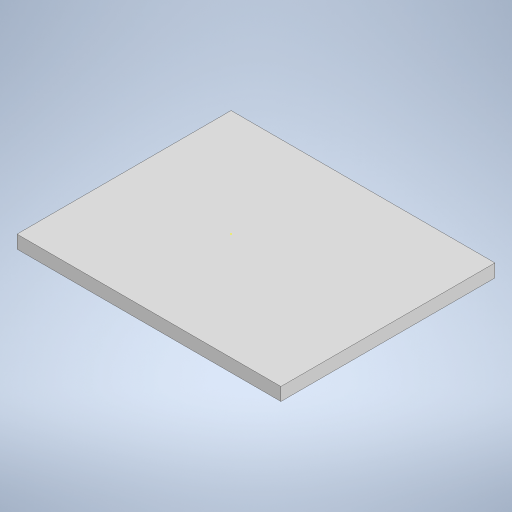
# Autodesk Inventor part: Base
Saved by Autodesk Inventor 2024 (Build 280153000, 153)
## iProperties
Created: 2023-10-07
Part Number: Base
Material: Generic
Document SubType Name: Modeling
Designer: chris
Density: 1 g/cm^3
Appearance: Default
Author: chris
Autodesk Inventor part; units mm, degrees
ref_plane "YZ Plane" through (0, 0, 0) normal (1, 0, 0) x (0, 1, 0)
ref_plane "XZ Plane" through (0, 0, 0) normal (0, 1, 0) x (-1, 0, 0)
ref_plane "XY Plane" through (0, 0, 0) normal (0, 0, 1) x (1, 0, 0)
sketch "Sketch1" plane through (0, 0, 0) normal (0, 1, 0) x (-1, 0, 0)
  line L0 (26.36, 26.36) -> (-26.36, 26.36)
  line L1 (-26.36, 26.36) -> (-26.36, -26.36)
  line L2 (-26.36, -26.36) -> (26.36, -26.36)
  line L3 (26.36, -26.36) -> (26.36, 26.36)
  line L4 (26.36, 26.36) -> (-26.36, -26.36) construction
  line L5 (-26.36, 26.36) -> (26.36, -26.36) construction
  line L6 (-26.36, -26.36) -> (-38.64, -26.36)
  line L7 (-38.64, -26.36) -> (-38.64, 26.36)
  line L8 (-38.64, 26.36) -> (-26.36, 26.36)
  line L9 (-26.36, 26.36) -> (-26.36, -26.36)
  point P0 (0, 0)
  dimension "d4" = 65
  dimension "d5" = 52.72
  constraints: 20 end point, 4 parallel, 3 perpendicular, 2 horizontal, 2 midpoint, 1 collinear
  measures "d4" distance between parallel lines of L3 L7
  measures "d5" distance between parallel lines of L8 L6
extrude "Extrusion1" add sketch "Sketch1" along normal blind 3.2
sketch "Sketch2" plane through (0, 3.2, 0) normal (0, 1, 0) x (1, 0, 0)
  point P0 (0, 0)
body "Solid1"
